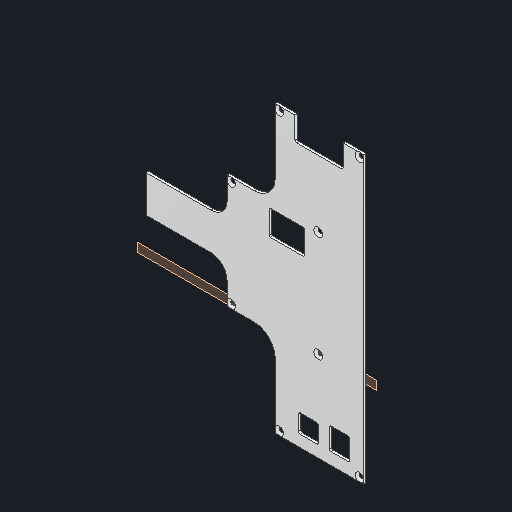
# Autodesk Inventor part: ceil
Saved by Autodesk Inventor 2023 (Build 270158000, 158)
## iProperties
Created: 2024-05-26
Part Number: ceil
Material: ABS Plastic
Document SubType Name: Modeling
Designer: szymo
Density: 1.06 g/cm^3
Appearance: Smooth - White
Mass: 19.0981 g
Surface Area: 253.991 cm^2
Volume: 18.0171 cm^3
Author: szymo
Autodesk Inventor part; units mm, degrees
ref_plane "YZ Plane" through (0, 0, 0) normal (1, 0, 0) x (0, 1, 0)
ref_plane "XZ Plane" through (0, 0, 0) normal (0, 1, 0) x (-1, 0, 0)
ref_plane "XY Plane" through (0, 0, 0) normal (0, 0, 1) x (1, 0, 0)
ref_plane "Work Plane1" through (-50.5, 0, 0) normal (0, 0, 1) x (1, 0, 0)
sketch "Sketch3" plane through (-50.5, 0, 0) normal (0, 0, 1) x (1, 0, 0)
  line L0 (0, 0) -> (135.5648, 0) projected
  line L1 (135.5648, 0) -> (135.5648, 5) projected
  line L2 (0, 5) -> (135.5648, 5) projected
  line L3 (0, 0) -> (0, 5) projected
  line L4 (0, 24) -> (50.5, 24) projected
  line L5 (0, 47) -> (50.5, 47) projected
  line L6 (0, 71) -> (135.5648, 71) projected
  line L7 (0, 71) -> (0, 66) projected
  line L8 (0, 66) -> (135.5648, 66) projected
  line L9 (135.5648, 71) -> (135.5648, 66) projected
  arc A0 (130.5648, 120.5) -> (131.5648, 119.5) centre (131.5648, 120.5) ccw projected
  line L10 (131.5648, 119.5) -> (134.5648, 119.5) projected
  arc A1 (134.5648, 119.5) -> (135.5648, 120.5) centre (134.5648, 120.5) ccw projected
  line L11 (135.5648, 124.5) -> (135.5648, 120.5) projected
  line L12 (135.5648, 124.5) -> (50.5, 124.5) projected
  line L13 (50.5, 124.5) -> (50.5, 123.5) projected
  line L14 (50.5, 123.5) -> (80.5, 123.5) projected
  line L15 (80.5, 123.5) -> (80.5, 120.5) projected
  arc A2 (80.5, 120.5) -> (81.5, 119.5) centre (81.5, 120.5) ccw projected
  line L16 (81.5, 119.5) -> (84.5, 119.5) projected
  arc A3 (84.5, 119.5) -> (85.5, 120.5) centre (84.5, 120.5) ccw projected
  line L17 (85.5, 123.5) -> (85.5, 120.5) projected
  line L18 (85.5, 123.5) -> (130.5648, 123.5) projected
  line L19 (130.5648, 123.5) -> (130.5648, 120.5) projected
  circle A4 centre (133.0648, 122) radius 1.75 projected
  circle A5 centre (83, 122) radius 1.75 projected
  line L20 (120.8148, 112) -> (120.8148, 123) projected
  line L21 (120.8148, 123) -> (94.8148, 123) projected
  line L22 (94.8148, 123) -> (94.8148, 112) projected
  line L23 (94.8148, 112) -> (120.8148, 112) projected
  arc A6 (131.5648, -48.5) -> (130.5648, -49.5) centre (131.5648, -49.5) ccw projected
  line L24 (130.5648, -52.5) -> (130.5648, -49.5) projected
  line L25 (85.5, -52.5) -> (130.5648, -52.5) projected
  line L26 (85.5, -52.5) -> (85.5, -49.5) projected
  arc A7 (85.5, -49.5) -> (84.5, -48.5) centre (84.5, -49.5) ccw projected
  line L27 (81.5, -48.5) -> (84.5, -48.5) projected
  arc A8 (81.5, -48.5) -> (80.5, -49.5) centre (81.5, -49.5) ccw projected
  line L28 (80.5, -52.5) -> (80.5, -49.5) projected
  line L29 (50.5, -52.5) -> (80.5, -52.5) projected
  line L30 (50.5, -53.5) -> (50.5, -52.5) projected
  line L31 (135.5648, -53.5) -> (50.5, -53.5) projected
  line L32 (135.5648, -53.5) -> (135.5648, -49.5) projected
  arc A9 (135.5648, -49.5) -> (134.5648, -48.5) centre (134.5648, -49.5) ccw projected
  line L33 (131.5648, -48.5) -> (134.5648, -48.5) projected
  circle A10 centre (133.0648, -51) radius 1.75 projected
  circle A11 centre (83, -51) radius 1.75 projected
  line L34 (95.5648, -45.8) -> (95.5648, -35.2) projected
  line L35 (106.8648, -35.2) -> (95.5648, -35.2) projected
  line L36 (106.8648, -35.2) -> (106.8648, -45.8) projected
  line L37 (95.5648, -45.8) -> (106.8648, -45.8) projected
  circle A12 centre (90.4898, -49.075) radius 1.675 projected
  circle A13 centre (124.5398, -49.075) radius 1.675 projected
  line L38 (126.3648, -33.5) -> (126.3648, -45.5) projected
  line L39 (126.3648, -45.5) -> (114.7648, -45.5) projected
  line L40 (114.7648, -45.5) -> (114.7648, -33.5) projected
  line L41 (114.7648, -33.5) -> (86.8648, -33.5) projected
  line L42 (86.8648, -33.5) -> (86.8648, -52.5) projected
  line L43 (86.8648, -52.5) -> (128.0648, -52.5) projected
  line L44 (128.0648, -52.5) -> (128.0648, -33.5) projected
  line L45 (128.0648, -33.5) -> (126.3648, -33.5) projected
  line L46 (126.3648, -32.7) -> (114.7648, -32.7) projected
  line L47 (114.7648, -32.7) -> (114.7648, -45.5) projected
  line L48 (114.7648, -45.5) -> (126.3648, -45.5) projected
  line L49 (126.3648, -45.5) -> (126.3648, -32.7) projected
  line L50 (80.5, -53.5) -> (135.5648, -53.5)
  line L51 (135.5648, -53.5) -> (135.5648, 124.5)
  line L52 (135.5648, 124.5) -> (80.5, 124.5)
  line L53 (80.5, 124.5) -> (80.5, -53.5)
  line L54 (0, 24) -> (80.5, 24)
  line L55 (80.5, 24) -> (80.5, 47)
  line L56 (80.5, 47) -> (0, 47)
  line L57 (0, 47) -> (0, 24)
  line L58 (80.5, 24) -> (50.5, 24)
  line L59 (50.5, 24) -> (50.5, 0)
  line L60 (50.5, 0) -> (80.5, 0)
  line L61 (80.5, 0) -> (80.5, 24)
  line L62 (50.5, 47) -> (80.5, 47)
  line L63 (80.5, 47) -> (80.5, 71)
  line L64 (80.5, 71) -> (50.5, 71)
  line L65 (50.5, 71) -> (50.5, 47)
  arc A14 (97.9124, 51.3) -> (98.0124, 51.4) centre (97.9124, 51.4) ccw projected
  line L66 (77.4124, 51.3) -> (97.9124, 51.3) projected
  arc A15 (77.3124, 51.4) -> (77.4124, 51.3) centre (77.4124, 51.4) ccw projected
  line L67 (77.3124, 65.9) -> (77.3124, 51.4) projected
  arc A16 (77.4124, 66) -> (77.3124, 65.9) centre (77.4124, 65.9) ccw projected
  line L68 (97.9124, 66) -> (77.4124, 66) projected
  arc A17 (98.0124, 65.9) -> (97.9124, 66) centre (97.9124, 65.9) ccw projected
  line L69 (98.0124, 51.4) -> (98.0124, 65.9) projected
  line L70 (96.2124, 64.1) -> (96.2124, 53.2) projected
  arc A18 (96.2124, 64.1) -> (95.9124, 64.4) centre (95.9124, 64.1) ccw projected
  line L71 (95.9124, 64.4) -> (95.8124, 64.4) projected
  line L72 (95.8124, 64.4) -> (95.3509, 64.95) projected
  line L73 (95.3509, 64.95) -> (94.9739, 64.95) projected
  line L74 (94.9739, 64.95) -> (94.5124, 64.4) projected
  line L75 (94.5124, 64.4) -> (90.8124, 64.4) projected
  line L76 (90.8124, 64.4) -> (90.8124, 64.75) projected
  line L77 (90.8124, 64.75) -> (89.5124, 64.75) projected
  line L78 (89.5124, 64.4) -> (89.5124, 64.75) projected
  line L79 (89.5124, 64.4) -> (85.8124, 64.4) projected
  line L80 (85.8124, 64.4) -> (85.8124, 64.75) projected
  line L81 (85.8124, 64.75) -> (84.5124, 64.75) projected
  line L82 (84.5124, 64.4) -> (84.5124, 64.75) projected
  line L83 (84.5124, 64.4) -> (80.8124, 64.4) projected
  line L84 (80.8124, 64.4) -> (80.3509, 64.95) projected
  line L85 (80.3509, 64.95) -> (79.9739, 64.95) projected
  line L86 (79.9739, 64.95) -> (79.5124, 64.4) projected
  line L87 (79.5124, 64.4) -> (79.4124, 64.4) projected
  arc A19 (79.4124, 64.4) -> (79.1124, 64.1) centre (79.4124, 64.1) ccw projected
  line L88 (79.1124, 64.1) -> (79.1124, 53.2) projected
  arc A20 (79.1124, 53.2) -> (79.4124, 52.9) centre (79.4124, 53.2) ccw projected
  line L89 (79.4124, 52.9) -> (79.5124, 52.9) projected
  line L90 (79.5124, 52.9) -> (79.9739, 52.35) projected
  line L91 (80.3509, 52.35) -> (79.9739, 52.35) projected
  line L92 (80.3509, 52.35) -> (80.8124, 52.9) projected
  line L93 (80.8124, 52.9) -> (84.5124, 52.9) projected
  line L94 (84.5124, 52.9) -> (84.5124, 52.55) projected
  line L95 (85.8124, 52.55) -> (84.5124, 52.55) projected
  line L96 (85.8124, 52.9) -> (85.8124, 52.55) projected
  line L97 (85.8124, 52.9) -> (89.5124, 52.9) projected
  line L98 (89.5124, 52.9) -> (89.5124, 52.55) projected
  line L99 (90.8124, 52.55) -> (89.5124, 52.55) projected
  line L100 (90.8124, 52.9) -> (90.8124, 52.55) projected
  line L101 (90.8124, 52.9) -> (94.5124, 52.9) projected
  line L102 (94.5124, 52.9) -> (94.9739, 52.35) projected
  line L103 (95.3509, 52.35) -> (94.9739, 52.35) projected
  line L104 (95.3509, 52.35) -> (95.8124, 52.9) projected
  line L105 (95.8124, 52.9) -> (95.9124, 52.9) projected
  arc A21 (95.9124, 52.9) -> (96.2124, 53.2) centre (95.9124, 53.2) ccw projected
  line L106 (78.1624, 55.75) -> (78.8624, 55.75) projected
  line L107 (78.8624, 55.75) -> (78.8624, 61.55) projected
  line L108 (78.1624, 61.55) -> (78.8624, 61.55) projected
  line L109 (78.1624, 61.55) -> (78.1624, 55.75) projected
  line L110 (97.1624, 61.55) -> (97.1624, 55.75) projected
  line L111 (96.4624, 61.55) -> (97.1624, 61.55) projected
  line L112 (96.4624, 55.75) -> (96.4624, 61.55) projected
  line L113 (96.4624, 55.75) -> (97.1624, 55.75) projected
  arc A22 (76.8124, 51.4) -> (77.4124, 50.8) centre (77.4124, 51.4) ccw
  line L114 (77.4124, 50.8) -> (97.9124, 50.8)
  arc A23 (97.9124, 50.8) -> (98.5124, 51.4) centre (97.9124, 51.4) ccw
  line L115 (98.5124, 51.4) -> (98.5124, 65.9)
  arc A24 (98.5124, 65.9) -> (97.9124, 66.5) centre (97.9124, 65.9) ccw
  line L116 (97.9124, 66.5) -> (77.4124, 66.5)
  arc A25 (77.4124, 66.5) -> (76.8124, 65.9) centre (77.4124, 65.9) ccw
  line L117 (76.8124, 65.9) -> (76.8124, 51.4)
  line L118 (95.0648, -34.7) -> (95.0648, -46.3)
  line L119 (95.0648, -46.3) -> (107.3648, -46.3)
  line L120 (107.3648, -46.3) -> (107.3648, -34.7)
  line L121 (107.3648, -34.7) -> (95.0648, -34.7)
  line L122 (114.2648, -45.5) -> (114.2648, -32.2)
  line L123 (114.2648, -32.2) -> (126.8648, -32.2)
  line L124 (126.8648, -32.2) -> (126.8648, -45.5)
  line L125 (126.3648, -46) -> (114.7648, -46)
  line L126 (92.8148, 110) -> (92.8148, 125)
  line L127 (92.8148, 125) -> (122.8148, 125)
  line L128 (122.8148, 125) -> (122.8148, 110)
  line L129 (122.8148, 110) -> (92.8148, 110)
  line L130 (114.2648, -45.5) -> (114.2648, -46)
  line L131 (114.2648, -46) -> (114.7648, -46)
  line L132 (126.3648, -46) -> (126.8648, -46)
  line L133 (126.8648, -46) -> (126.8648, -45.5)
  line L134 (0, 47) -> (0, 42.5) projected
  line L135 (0, 42.5) -> (50.5, 42.5) projected
  line L136 (50.5, 47) -> (50.5, 42.5) projected
  line L137 (50.5, 24) -> (50.5, 28.5) projected
  line L138 (0, 28.5) -> (50.5, 28.5) projected
  line L139 (0, 24) -> (0, 28.5) projected
  circle A26 centre (105.3205, 68.5) radius 1.75 projected
  circle A27 centre (53, 68.5) radius 1.75 projected
  circle A28 centre (105.3205, 2.5) radius 1.75 projected
  circle A29 centre (53, 2.5) radius 1.75 projected
  point P0 (122.8148, 124.5)
  point P1 (92.8148, 124.5)
  point P2 (80.5, 0)
  point P3 (0, 44)
  point P4 (50.5, 44)
  point P5 (122.8148, 124.5)
  point P6 (122.8148, 123.5)
  point P7 (92.8148, 123.5)
  point P8 (92.8148, 124.5)
  point P9 (50.5, 66)
  point P10 (50.5, 5)
  point P11 (80.5, 66)
  point P12 (80.5, 5)
  point P13 (50.5, 27)
  point P14 (0, 27)
  dimension "d16" = 0.5
  dimension "d17" = 0.5
  dimension "d18" = 0.5
  dimension "d19" = 0.5
  dimension "d20" = 2
  constraints: 72 end point, 9 parallel, 8 point on circle, 6 perpendicular, 5 point on line, 4 centre point, 4 horizontal, 2 collinear, 1 vertical, 15 other
  measures "d16" distance between parallel lines of L67 L117
  measures "d17" distance between parallel lines of L34 L118
  measures "d18" distance between parallel lines of L47 L122
  measures "d19" distance between parallel lines of L39 L125
  measures "d20" distance between parallel lines of L22 L126
extrude "Extrusion2" add sketch "Sketch3" along normal blind 1.5 contours L59 L2 L53 L0 | L53 L2 L1 L0 | L0 L51 A9 L33 A6 L24 L25 L44 L45 L124 L123 L122 L41 L42 L26 A7 L27 A8 L53 | L59 L54 L53 L2 | A8 L27 A7 L26 L25 L24 A6 L33 A9 L32 L31 L53 L28 | L53 L114 A23 L115 A24 L8 L51 L2 | L137 L138 L57 L135 L136 L56 L53 L54 | L4 L57 L138 L137 | L8 A24 L116 L53 L6 L9 | L56 L65 L8 A25 L117 A22 L114 L53 | L6 L53 A2 L16 A3 L17 L18 L126 L129 L128 L19 A0 L10 A1 L51 | L136 L135 L57 L5 | L53 L116 A25 L8 L65 L6 | A1 L10 A0 L19 L18 L128 L12 L11 | L15 L53 L12 L126 L18 L17 A3 L16 A2 | L42 L41 L122 L130 L131 L125 L132 L133 L124 L45 L44 L25 | A4 | A5 | A10 | A11 | A12 | A13 | A26 | A27 | A28 | A29
fillet "Fillet2" radius 1 10 edges at (44.5648, -46.3, 0.75) (44.5648, -34.7, 0.75) (56.8648, -34.7, 0.75) (56.8648, -46.3, 0.75) (63.7648, -46, 0.75) (63.7648, -32.2, 0.75) (76.3648, -32.2, 0.75) (76.3648, -46, 0.75) (42.3148, 110, 0.75) (72.3148, 110, 0.75)
fillet "Fillet3" radius 13 2 edges at (30, 0, 0.75) (30, 71, 0.75)
sketch "Sketch4" plane through (-50.5, 0, 1.5) normal (0, 0, 1) x (1, 0, 0)
  arc A0 (131.5648, -48.5) -> (130.5648, -49.5) centre (131.5648, -49.5) ccw projected
  line L0 (130.5648, -52.5) -> (130.5648, -49.5) projected
  line L1 (85.5, -52.5) -> (130.5648, -52.5) projected
  line L2 (85.5, -52.5) -> (85.5, -49.5) projected
  arc A1 (85.5, -49.5) -> (84.5, -48.5) centre (84.5, -49.5) ccw projected
  line L3 (81.5, -48.5) -> (84.5, -48.5) projected
  arc A2 (81.5, -48.5) -> (80.5, -49.5) centre (81.5, -49.5) ccw projected
  line L4 (80.5, -52.5) -> (80.5, -49.5) projected
  line L5 (50.5, -52.5) -> (80.5, -52.5) projected
  line L6 (50.5, -53.5) -> (50.5, -52.5) projected
  line L7 (135.5648, -53.5) -> (50.5, -53.5) projected
  line L8 (135.5648, -53.5) -> (135.5648, -49.5) projected
  arc A3 (135.5648, -49.5) -> (134.5648, -48.5) centre (134.5648, -49.5) ccw projected
  line L9 (131.5648, -48.5) -> (134.5648, -48.5) projected
  circle A4 centre (133.0648, -51) radius 1.75 projected
  circle A5 centre (83, -51) radius 1.75 projected
  arc A6 (130.5648, 120.5) -> (131.5648, 119.5) centre (131.5648, 120.5) ccw projected
  line L10 (131.5648, 119.5) -> (134.5648, 119.5) projected
  arc A7 (134.5648, 119.5) -> (135.5648, 120.5) centre (134.5648, 120.5) ccw projected
  line L11 (135.5648, 124.5) -> (135.5648, 120.5) projected
  line L12 (135.5648, 124.5) -> (50.5, 124.5) projected
  line L13 (50.5, 124.5) -> (50.5, 123.5) projected
  line L14 (50.5, 123.5) -> (80.5, 123.5) projected
  line L15 (80.5, 123.5) -> (80.5, 120.5) projected
  arc A8 (80.5, 120.5) -> (81.5, 119.5) centre (81.5, 120.5) ccw projected
  line L16 (81.5, 119.5) -> (84.5, 119.5) projected
  arc A9 (84.5, 119.5) -> (85.5, 120.5) centre (84.5, 120.5) ccw projected
  line L17 (85.5, 123.5) -> (85.5, 120.5) projected
  line L18 (85.5, 123.5) -> (130.5648, 123.5) projected
  line L19 (130.5648, 123.5) -> (130.5648, 120.5) projected
  circle A10 centre (133.0648, 122) radius 1.75 projected
  circle A11 centre (83, 122) radius 1.75 projected
  line L20 (0, 71) -> (135.5648, 71) projected
  line L21 (0, 71) -> (0, 66) projected
  line L22 (0, 66) -> (135.5648, 66) projected
  line L23 (135.5648, 71) -> (135.5648, 66) projected
  line L24 (0, 0) -> (135.5648, 0) projected
  line L25 (135.5648, 0) -> (135.5648, 5) projected
  line L26 (0, 5) -> (135.5648, 5) projected
  line L27 (0, 0) -> (0, 5) projected
  line L28 (0, 24) -> (50.5, 24) projected
  line L29 (0, 47) -> (50.5, 47) projected
  line L30 (0, 47) -> (0, 42.5) projected
  line L31 (0, 42.5) -> (50.5, 42.5) projected
  line L32 (50.5, 47) -> (50.5, 42.5) projected
  line L33 (50.5, 24) -> (50.5, 28.5) projected
  line L34 (0, 28.5) -> (50.5, 28.5) projected
  line L35 (0, 24) -> (0, 28.5) projected
  circle A12 centre (105.3205, 68.5) radius 1.75 projected
  circle A13 centre (53, 68.5) radius 1.75 projected
  circle A14 centre (105.3205, 2.5) radius 1.75 projected
  circle A15 centre (53, 2.5) radius 1.75 projected
  point P0 (50.5, 0)
  point P1 (107.3205, 68.5)
  point P2 (107.3205, 2.5)
  point P3 (0, 44)
  point P4 (50.5, 44)
  point P5 (50.5, 27)
  point P6 (0, 27)
  constraints: 4 coincident
hole "Hole2" at (32.5, -51, 1.5) at (82.5648, -51, 1.5) at (82.5648, 122, 1.5) at (32.5, 122, 1.5) at (56.8205, 68.5, 1.5) at (56.8205, 2.5, 1.5) at (2.5, 2.5, 1.5) at (2.5, 68.5, 1.5) direction (0, 0, -1) diameter 2.9 end through all countersink diameter 5.5 countersink angle 90 clearance for "Countersunk Flat Head Screw ISO 2009/7046" size "M2.5" standard "ISO"
fillet "Fillet4" radius 10 2 edges at (0, 24, 0.75) (0, 47, 0.75)
body "Solid2"
